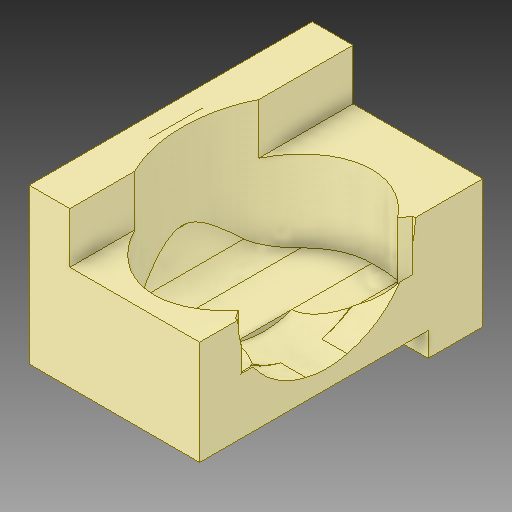
# Autodesk Inventor part: tip_plate
Saved by Autodesk Inventor 2019 (Build 230136000, 136)
## iProperties
Created: 2024-08-26
Part Number: tip_plate
Material: Nylon 6/6
Document SubType Name: Modeling
Designer: nic
Density: 1.13 g/cm^3
Appearance: Nylon 6
Mass: 1.62597 g
Surface Area: 16.0059 cm^2
Volume: 1.62597 cm^3
Author: nic
Autodesk Inventor part; units mm, degrees
ref_plane "YZ Plane" through (0, 0, 0) normal (1, 0, 0) x (0, 1, 0)
ref_plane "XZ Plane" through (0, 0, 0) normal (0, 1, 0) x (-1, 0, 0)
ref_plane "XY Plane" through (0, 0, 0) normal (0, 0, 1) x (1, 0, 0)
sketch "Skizze2" plane through (0, 0, 0) normal (0, 0, 1) x (1, 0, 0)
  line L0 (-6.1986, -18.7338) -> (-6.1496, -19.0193) construction
  line L1 (-3.0691, -22.5033) -> (-3.0261, -22.5027) construction
  line L2 (7.5424, -18.0048) -> (7.3049, -18.5009) construction
  line L3 (6.2261, -17.7959) -> (6.1028, -18.1348) construction
  line L4 (0, -22.5023) -> (0, -12.3023) construction
  line L5 (0, -17.4023) -> (-5, -17.4023) construction
  line L6 (-5, -17.4023) -> (5, -17.4023) construction
  line L7 (-5.9231, -17.4238) -> (-8.4231, -17.4238) construction
  line L8 (0, -22.5023) -> (0, -24.5023) construction
  line L9 (5, -20.0874) -> (5, -24.5033)
  line L10 (5, -24.5033) -> (-8.4231, -24.5033)
  line L11 (-8.4231, -24.5033) -> (-8.4231, -12.3033)
  line L12 (-3.846, -22.5023) -> (0, -22.5023) construction
  arc A0 (-6.1496, -19.0193) -> (-5.4111, -21.511) centre (4.6922, -17.161) ccw construction
  arc A1 (-5.4111, -21.511) -> (-3.846, -22.5023) centre (-3.9035, -20.8619) ccw construction
  arc A2 (-6.6716, -12.3033) -> (-6.1496, -19.0193) centre (29.9153, -12.8378) ccw construction
  line L13 (3.1841, -21.5122) -> (2.6713, -21.7923) projected
  line L14 (4.8434, -19.8809) -> (4.6255, -20.1379) projected
  arc A3 (0, -22.5023) -> (3.1841, -21.5122) centre (0, -16.8873) ccw construction
  arc A4 (3.1841, -21.5122) -> (5, -19.6961) centre (0.9978, -17.5102) ccw construction
  arc A5 (3.289, -21.6827) -> (5, -20.0874) centre (0.9978, -17.5102) ccw
  arc A6 (0, -22.7023) -> (3.289, -21.6827) centre (0, -16.8873) ccw
  line L15 (0, -22.7023) -> (-3.8426, -22.7023)
  arc A7 (-5.5948, -21.5901) -> (-3.8426, -22.7023) centre (-3.9035, -20.8619) ccw
  arc A8 (-6.3468, -19.0531) -> (-5.5948, -21.5901) centre (4.6922, -17.161) ccw
  arc A9 (-6.8716, -12.3004) -> (-6.3468, -19.0531) centre (29.9153, -12.8378) ccw
  line L16 (-8.4231, -12.3033) -> (-6.8717, -12.3033)
  point P0 (0, 0)
  dimension "d14" = 0.2
  constraints: 22 end point, 21 point on circle, 10 centre point, 5 tangent, 4 horizontal, 2 parallel, 2 vertical, 1 midpoint, 1 perpendicular, 1 point on line, 4 other
  measures "d14" radial gap between concentric circles of A0 A8
extrude "Extrusion2" add sketch "Skizze2" along normal mid plane 20
sketch "Skizze3" plane through (5, -24.5033, 10) normal (1, 0, 0) x (0, 0, -1)
  circle A0 centre (10, 7.9958) radius 6.5945
  point P0 (10, 24.5033)
  constraints: 1 centre point
extrude "Extrusion3" cut sketch "Skizze3" against normal blind 5
sketch "Skizze4" plane through (-8.4231, -24.5033, 10) normal (0, -1, 0) x (1, 0, 0)
  line L0 (7.2368, -0.8632) -> (6.8535, -0.9732) projected
  line L1 (10.5566, -1.1946) -> (10.2147, -1.0518) projected
  line L2 (4.42, -17.4729) -> (4.7168, -17.757) projected
  line L3 (11.7618, -18.0665) -> (12.0769, -17.8039) projected
  line L4 (1.6881, -10.5104) -> (1.6815, -10.0518) projected
  line L5 (1.8037, -8.2282) -> (1.8886, -7.7318) projected
  line L6 (2.5827, -5.3733) -> (2.4034, -5.8192) projected
  line L7 (3.9903, -3.0146) -> (4.2787, -2.6949) projected
  line L8 (8.0017, -0.745) -> (8.4176, -0.7333) projected
  line L9 (8.4182, -19.2683) -> (8.096, -19.2621) projected
  line L10 (2.6734, -14.8449) -> (2.5089, -14.4448) projected
  line L11 (1.6881, -10.5104) -> (1.6815, -10.0518) projected
  line L12 (2.4067, -5.8226) -> (2.2455, -6.2815) projected
  ellipse E0 centre (8.4231, -10) end of major axis (8.4231, -0.7333) minor radius 6.7401 construction
  line L13 (8.4231, -20) -> (8.4231, 0) projected
  ellipse E1 centre (8.4231, -10) end of major axis (8.4231, -0.4333) minor radius 7.0401 (13.4231, -3.2652) -> (13.4231, -16.7348) ccw
  line L14 (13.4231, -20) -> (13.4231, 0) projected
  line L15 (13.4231, -16.7348) -> (13.4231, -3.2652)
  line L16 (13.4231, -20) -> (0, -20)
  line L17 (0, -20) -> (0, 0)
  line L18 (0, 0) -> (13.4231, 0)
  line L19 (13.4231, 0) -> (13.4231, -20)
  constraints: 10 end point, 2 parallel, 2 point on line, 1 coincident, 1 horizontal, 1 perpendicular, 1 vertical, 7 other
extrude "Extrusion4" add sketch "Skizze4" against normal up to surface (12.2 mm away) contours L16 L17 L18 L13 E1 | L13 E1 L14 L16 | L13 L18 L14 E1
sketch "Skizze5" plane through (5, -24.5033, 10) normal (1, 0, 0) x (0, 0, -1)
  ellipse E0 centre (10, 8.2175) end of major axis (16.9904, 8.2175) minor radius 6.7992
  point P0 (10, 24.5033)
  constraints: 2 other
extrude "Extrusion5" cut sketch "Skizze5" against normal blind 2
sketch "Skizze6" plane through (0, 0, -10) normal (0, 0, -1) x (-1, 0, 0)
  line L0 (-5, -12.3033) -> (-5, -20.0874) projected
  line L1 (-5, -12.3033) -> (5.2227, -12.3033)
  line L2 (5.2227, -12.3033) -> (5.2227, -16.3033)
  line L3 (5.2227, -16.3033) -> (-5, -16.3033)
  line L4 (-5, -16.3033) -> (-5, -12.3033)
  point P0 (0, 0)
  dimension "d24" = 4
  constraints: 8 end point, 2 parallel, 1 horizontal, 1 perpendicular
  measures "d24" distance of L1.end L2.end
extrude "Extrusion6" cut sketch "Skizze6" against normal through all
sketch "Skizze7" plane through (0, 0, -10) normal (0, 0, -1) x (-1, 0, 0)
  line L0 (-5, -24.5033) -> (-5, -16.3033) projected
  line L1 (-5, -16.3033) -> (5.1, -16.3033)
  line L2 (5.1, -26.4033) -> (-5, -26.4033)
  line L3 (-5, -26.4033) -> (-5, -16.3033)
  line L4 (-5, -16.3033) -> (8.4231, -16.3033)
  line L5 (8.4231, -16.3033) -> (8.4231, -26.4033)
  line L6 (8.4231, -26.4033) -> (-5, -26.4033)
  line L7 (-5, -26.4033) -> (-5, -16.3033)
  line L8 (8.4231, -24.5033) -> (-5, -24.5033) projected
  line L9 (-5, -24.5033) -> (8.4231, -24.5033)
  point P0 (0, 0)
  constraints: 16 end point, 4 equal length, 2 horizontal, 1 perpendicular
extrude "Extrusion7" add sketch "Skizze7" against normal blind 2 contours L8 L5 L6 L2 L3
sketch "Skizze8" plane through (0, 0, -10) normal (0, 0, -1) x (-1, 0, 0)
  line L0 (5.2227, -16.3033) -> (-5, -16.3033) projected
  line L1 (-5, -26.4033) -> (-5, -16.3033) projected
  line L2 (-5, -26.4033) -> (8.4231, -26.4033) projected
  line L3 (8.4231, -26.4033) -> (8.4231, -12.3033) projected
  line L4 (8.4231, -12.3033) -> (5.2227, -12.3033) projected
  line L5 (5.2227, -12.3033) -> (5.2227, -16.3033) projected
  point P0 (0, 0)
extrude "Extrusion8" add sketch "Skizze8" along normal blind 2.3
sketch "Skizze9" plane through (-6.8717, -12.3033, 2.0803) normal (0, 1, 0) x (1, 0, 0)
  ellipse E0 centre (6.8717, 2.0803) end of major axis (6.8717, -7.4864) minor radius 7.0401 (1.649, -4.3348) -> (11.6779, -4.9101) ccw projected
  ellipse E1 centre (6.8717, 2.0803) end of major axis (6.8717, -7.4864) minor radius 7.0401 (0, 0) -> (1.649, -4.3348) ccw projected
  line L0 (0, 4.1607) -> (0, 0) projected
  ellipse E2 centre (6.8717, 2.0803) end of major axis (6.8717, -7.4864) minor radius 7.0401 (1.649, 8.4955) -> (0, 4.1607) ccw projected
  ellipse E3 centre (6.8717, 2.0803) end of major axis (6.8717, -7.4864) minor radius 7.0401 (11.6779, 9.0708) -> (1.649, 8.4955) ccw projected
  arc A0 (11.8717, -5.235) -> (11.5183, -5.1066) centre (11.6717, -5.235) ccw projected
  arc A1 (11.5183, 9.2672) -> (11.8717, 9.3957) centre (11.6717, 9.3957) ccw projected
  ellipse E4 centre (6.8717, 2.0803) end of major axis (6.8717, 10.647) minor radius 6.3555 (11.1965, 8.3578) -> (11.1965, -4.1971) ccw
  line L1 (6.8717, -0.1806) -> (6.8717, 4.3413) construction
  line L2 (6.8716, 11.647) -> (6.8716, -7.4864) construction
  ellipse E5 centre (6.8717, 2.0803) end of major axis (6.8717, 11.647) minor radius 7.0401 (11.6779, 9.0708) -> (11.6779, -4.9101) ccw
  line L3 (11.6779, -4.9101) -> (11.1965, -4.1971)
  line L4 (11.8717, 9.0708) -> (11.6779, 9.0708) construction
  line L5 (11.6779, 9.0708) -> (11.1965, 8.3578)
  constraints: 5 end point, 2 coincident, 2 vertical, 13 other
extrude "Extrusion9" add sketch "Skizze9" against normal up to surface (10.399 mm away) contours E1 L0 E2 E3 L5 E4 L3 E0
sketch "Skizze10" plane through (-8.4231, -12.3033, 10) normal (0, 1, 0) x (1, 0, 0)
  ellipse E0 centre (8.4231, 10) end of major axis (8.4231, 1.4333) minor radius 6.3555 (12.7479, 16.2774) -> (12.7479, 3.7226) ccw projected
  ellipse E1 centre (8.4231, 10) end of major axis (8.4231, 0.4333) minor radius 7.0401 (3.2004, 3.5848) -> (13.2294, 3.0096) ccw projected
  ellipse E2 centre (8.4231, 10) end of major axis (8.4231, 0.4333) minor radius 7.0401 (13.2294, 16.9904) -> (3.2004, 16.4152) ccw projected
  line L0 (13.4231, 16.9904) -> (13.2294, 16.9904) projected
  line L1 (13.4231, 22.3) -> (13.4231, 16.9904) projected
  line L2 (3.2004, 22.3) -> (13.4231, 22.3) projected
  line L3 (3.2004, 22.3) -> (3.2004, 16.4152) projected
  ellipse E3 centre (8.4231, 10) end of major axis (8.4231, 18.5667) minor radius 6.3555 (3.2004, 5.1184) -> (3.2004, 14.8816) ccw
  ellipse E4 centre (8.4231, 10) end of major axis (8.4231, 19.5667) minor radius 7.0401 (3.2004, 3.5848) -> (3.2004, 16.4152) ccw
  line L4 (3.2004, 3.5848) -> (3.2004, 16.4152)
  constraints: 2 coincident, 2 end point, 2 point on line, 1 vertical, 12 other
extrude "Extrusion10" cut sketch "Skizze10" against normal up to surface (4 mm away) contours E0 L4 E2 E4 E1 E3
